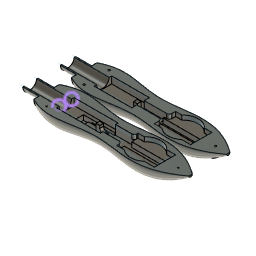
Fork V2 Fusion360 (Autodesk Fusion 360 design; units mm, degrees)
Autodesk Fusion 360 part; units mm, degrees
sketch "Sketch1" plane through (0, 0, 0) normal (0, 0, 1) x (1, 0, 0)
  line L0 (15.0107, 0) -> (130.0107, 0)
  line L1 (15.0107, 10.1439) -> (15.0107, 0)
  line L2 (130.0107, 1.3892) -> (130.0107, 0)
  spline S0 degree 5 poles (15.0107, 10.1439) (17.1655, 11.3215) (21.4632, 13.2587) (27.8735, 14.9106) (36.3471, 14.9335) (46.8266, 13.042) (57.2393, 11.1221) (67.6884, 10.6548) (78.3704, 11.8963) (89.578, 13.6649) (101.6455, 14.0909) (112.252, 11.6814) (120.8621, 7.5393) (126.9099, 3.6304) (130.0107, 1.3892) knots 0 0 0 0 0 0 0.1 0.2 0.3 0.4 0.5 0.6 0.7 0.8 0.9 1 1 1 1 1 1
  line L3 (5.0608, 4.7061) -> (24.9606, 15.5816)
  line L4 (117.8706, 10.1641) -> (142.1507, -7.3857)
  point P0 (63.5697, 11.0506)
  dimension "d2" = 115
  constraint horizontal L0
  constraint perpendicular L0 L1
  constraint perpendicular L0 L2
  constraint midpoint L1.start L3
  constraint midpoint L2.start L4
  measures "d2" distance of L0.start L0.end
revolve "Revolve1" add sketch "Sketch1" angle 360 about axis through (15.0107, 0, 0) along (1, 0, 0) makes body 1
sketch "Sketch2" plane through (0, 0, 0) normal (0, 0, 1) x (1, 0, 0)
sketch "Sketch3" plane through (15.0107, 0, 0) normal (-1, 0, 0) x (0, -1, 0)
  circle A0 centre (0, 0) radius 10.1439
  circle A1 centre (0, 0) radius 5
  circle A2 centre (0, 0) radius 6
  constraint coincident A0.centre A1.centre
extrude "Extrude1" add sketch "Sketch3" along normal blind 15 contours A2 bodies 1
extrude "Extrude2" cut 1 faces at (15.0107, 0.3379, -0.3642) along direction (1, 0, 0) blind 15 on bodies 1 bodies 1
split "Split1" by plane through (0, 0, 0) normal (0, 0, 1) bodies 1 makes body 2 at (53.0007, -11.0797, 4.6705)
move_body "Move1" bodies 2 to x (1, 0, 0) y (0, 1, 0) z (0, 0, 1) at (0, 0, 45)
sketch "Sketch4" plane through (0, 0, 0) normal (0, 0, 1) x (-1, 0, 0)
  line L0 (-15.0107, -6) -> (-0.0107, -6)
  line L1 (-0.0107, -6) -> (-0.0107, -5)
  line L2 (-0.0107, -5) -> (-30.0107, -5)
  line L3 (-30.0107, 5) -> (-0.0107, 5)
  line L4 (-0.0107, 5) -> (-0.0107, 6)
  line L5 (-0.0107, 6) -> (-15.0107, 6)
  line L6 (-15.0107, 6) -> (-15.0107, 10.1439)
  spline S0 degree 3 poles (-15.0107, 10.1439) (-17.2758, 11.3818) (-19.6235, 12.392) (-24.4058, 13.8233) (-26.7334, 14.2535) (-33.8193, 14.8563) (-38.417, 14.3623) (-51.6253, 12.321) (-59.2846, 10.4294) (-77.5088, 11.6941) (-83.806, 12.8904) (-95.9051, 13.7775) (-101.6068, 13.6874) (-114.9368, 10.4942) (-122.1312, 7.0845) (-130.0107, 1.3892) knots -19.403792 -19.403792 -19.403792 -19.403792 -17.868163 -17.868163 -16.437307 -16.437307 -13.646252 -13.646252 -8.493414 -8.493414 -5.456897 -5.456897 -2.916676 -2.916676 0 0 0 0
  line L7 (-130.0107, 1.3892) -> (-130.0107, -1.3892)
  spline S1 degree 5 poles (-15.0107, -10.1439) (-17.1655, -11.3215) (-21.4632, -13.2587) (-27.8735, -14.9106) (-36.3471, -14.9335) (-46.8266, -13.042) (-57.2393, -11.1221) (-67.6884, -10.6548) (-78.3704, -11.8963) (-89.578, -13.6649) (-101.6455, -14.0909) (-112.252, -11.6814) (-120.8621, -7.5393) (-126.9099, -3.6304) (-130.0107, -1.3892) knots 0 0 0 0 0 0 0.1 0.2 0.3 0.4 0.5 0.6 0.7 0.8 0.9 1 1 1 1 1 1
  line L8 (-15.0107, -10.1439) -> (-15.0107, -6)
move_body "Move2" bodies 2 to x (1, 0, 0) y (0, 1, 0) z (0, 0, 1) at (0, 65, 0)
sketch "Sketch5" plane through (0, 0, 0) normal (0, 0, 1) x (-1, 0, 0)
  line L0 (-30, -6) -> (-60, -6)
  line L1 (-60, -6) -> (-60, 6)
  line L2 (-60, 6) -> (-30, 6)
  line L3 (-30, 6) -> (-30, -6)
  constraint horizontal L0
  constraint vertical L1
  constraint horizontal L2
  constraint vertical L3
extrude "Extrude3" cut sketch "Sketch5" against normal blind 5.5 bodies 1
sketch "Sketch6" plane through (0, 0, 0) normal (0, 0, 1) x (1, 0, 0)
sketch "Sketch7" plane through (0, 0, -5.5) normal (0, 0, 1) x (-1, 0, 0)
  line L0 (-30, 6) -> (-60, 6)
  line L1 (-60, 6) -> (-60, -6)
  line L2 (-60, -6) -> (-30, -6)
  line L3 (-30, -6) -> (-30, 6)
  line L4 (-57, -1.5) -> (-59, -1.5)
  line L5 (-59, -1.5) -> (-59, 1.5)
  line L6 (-59, 1.5) -> (-57, 1.5)
  line L7 (-57, 1.5) -> (-57, -1.5)
  constraint horizontal L4
  constraint vertical L5
  constraint horizontal L6
  constraint vertical L7
extrude "Extrude4" add sketch "Sketch7" along normal blind 4 contours L4 L5 L6 L7 bodies 1
sketch "Sketch8" plane through (0, 0, 0) normal (0, 0, 1) x (-1, 0, 0)
  line L0 (-30, -5) -> (-30, -6)
  line L1 (-30, -6) -> (-60, -6)
  line L2 (-60, -6) -> (-60, 6)
  line L3 (-60, 6) -> (-30, 6)
  line L4 (-30, 6) -> (-30, 5)
  line L5 (-30, 5) -> (-0.0107, 5)
  line L6 (-0.0107, 5) -> (-0.0107, 6)
  line L7 (-0.0107, 6) -> (-15.0107, 6)
  line L8 (-15.0107, 6) -> (-15.0107, 10.1439)
  spline S0 degree 3 poles (-15.0107, 10.1439) (-17.2758, 11.3818) (-19.6235, 12.392) (-24.4058, 13.8233) (-26.7334, 14.2535) (-33.8193, 14.8563) (-38.417, 14.3623) (-51.6253, 12.321) (-59.2846, 10.4294) (-77.5088, 11.6941) (-83.806, 12.8904) (-95.9051, 13.7775) (-101.6068, 13.6874) (-114.9368, 10.4942) (-122.1312, 7.0845) (-130.0107, 1.3892) knots -19.403792 -19.403792 -19.403792 -19.403792 -17.868163 -17.868163 -16.437307 -16.437307 -13.646252 -13.646252 -8.493414 -8.493414 -5.456897 -5.456897 -2.916676 -2.916676 0 0 0 0
  line L9 (-130.0107, 1.3892) -> (-130.0107, -1.3892)
  spline S1 degree 5 poles (-15.0107, -10.1439) (-17.1655, -11.3215) (-21.4632, -13.2587) (-27.8735, -14.9106) (-36.3471, -14.9335) (-46.8266, -13.042) (-57.2393, -11.1221) (-67.6884, -10.6548) (-78.3704, -11.8963) (-89.578, -13.6649) (-101.6455, -14.0909) (-112.252, -11.6814) (-120.8621, -7.5393) (-126.9099, -3.6304) (-130.0107, -1.3892) knots 0 0 0 0 0 0 0.1 0.2 0.3 0.4 0.5 0.6 0.7 0.8 0.9 1 1 1 1 1 1
  line L10 (-15.0107, -10.1439) -> (-15.0107, -6)
  line L11 (-15.0107, -6) -> (-0.0107, -6)
  line L12 (-0.0107, -6) -> (-0.0107, -5)
  line L13 (-0.0107, -5) -> (-30, -5)
  line L14 (-60, -3) -> (-85, -3)
  line L15 (-85, -3) -> (-85, 3)
  line L16 (-85, 3) -> (-60, 3)
  line L17 (-60, 3) -> (-60, -3)
  constraint horizontal L14
  constraint vertical L15
  constraint horizontal L16
  constraint vertical L17
  constraint coincident L2 L14.start
extrude "Extrude5" cut sketch "Sketch8" against normal blind 2.5 contours L2 L14 L15 L16 L17 bodies 1
extrude "Extrude6" add 1 faces at (57.6667, 0.5, -1.5) along direction (0, 0, 1) blind 1 on bodies 1 bodies 1
sketch "Sketch9" plane through (0, 0, -5.5) normal (0, 0, 1) x (-1, 0, 0)
  line L0 (-57, 1.5) -> (-57, -1.5)
  line L1 (-57, -1.5) -> (-59, -1.5)
  line L2 (-59, -1.5) -> (-59, 1.5)
  line L3 (-59, 1.5) -> (-57, 1.5)
  line L4 (-30, 6) -> (-60, 6)
  line L5 (-60, 6) -> (-60, -6)
  line L6 (-60, -6) -> (-30, -6)
  line L7 (-30, -6) -> (-30, 6)
extrude "Extrude8" add 1 faces at (57, 0.5, -2.1667) along direction (-1, 0, 0) blind 2 on bodies 1 bodies 1
sketch "Sketch10" plane through (0, 0, 0) normal (0, 0, 1) x (-1, 0, 0)
  line L0 (-85, 3) -> (-60, 3)
  line L1 (-60, 3) -> (-60, 6)
  line L2 (-60, 6) -> (-30, 6)
  line L3 (-30, 6) -> (-30, 5)
  line L4 (-30, 5) -> (-0.0107, 5)
  line L5 (-0.0107, 5) -> (-0.0107, 6)
  line L6 (-0.0107, 6) -> (-15.0107, 6)
  line L7 (-15.0107, 6) -> (-15.0107, 10.1439)
  spline S0 degree 3 poles (-15.0107, 10.1439) (-17.2758, 11.3818) (-19.6235, 12.392) (-24.4058, 13.8233) (-26.7334, 14.2535) (-33.8193, 14.8563) (-38.417, 14.3623) (-51.6253, 12.321) (-59.2846, 10.4294) (-77.5088, 11.6941) (-83.806, 12.8904) (-95.9051, 13.7775) (-101.6068, 13.6874) (-114.9368, 10.4942) (-122.1312, 7.0845) (-130.0107, 1.3892) knots -19.403792 -19.403792 -19.403792 -19.403792 -17.868163 -17.868163 -16.437307 -16.437307 -13.646252 -13.646252 -8.493414 -8.493414 -5.456897 -5.456897 -2.916676 -2.916676 0 0 0 0
  line L8 (-130.0107, 1.3892) -> (-130.0107, -1.3892)
  spline S1 degree 5 poles (-15.0107, -10.1439) (-17.1655, -11.3215) (-21.4632, -13.2587) (-27.8735, -14.9106) (-36.3471, -14.9335) (-46.8266, -13.042) (-57.2393, -11.1221) (-67.6884, -10.6548) (-78.3704, -11.8963) (-89.578, -13.6649) (-101.6455, -14.0909) (-112.252, -11.6814) (-120.8621, -7.5393) (-126.9099, -3.6304) (-130.0107, -1.3892) knots 0 0 0 0 0 0 0.1 0.2 0.3 0.4 0.5 0.6 0.7 0.8 0.9 1 1 1 1 1 1
  line L9 (-15.0107, -10.1439) -> (-15.0107, -6)
  line L10 (-15.0107, -6) -> (-0.0107, -6)
  line L11 (-0.0107, -6) -> (-0.0107, -5)
  line L12 (-0.0107, -5) -> (-30, -5)
  line L13 (-30, -5) -> (-30, -6)
  line L14 (-30, -6) -> (-60, -6)
  line L15 (-60, -6) -> (-60, -3)
  line L16 (-60, -3) -> (-85, -3)
  line L17 (-85, -3) -> (-85, 3)
  line L18 (-80, -8) -> (-109, -8)
  line L19 (-109, -8) -> (-109, 9)
  line L20 (-109, 9) -> (-80, 9)
  line L21 (-80, 9) -> (-80, -8)
  dimension "d21" = 29
  dimension "d22" = 17
  constraint horizontal L18
  constraint vertical L19
  constraint horizontal L20
  constraint vertical L21
  measures "d21" distance of L18.start L18.end
  measures "d22" distance of L18.end L19.end
extrude "Extrude9" cut sketch "Sketch10" against normal blind 3.5 contours L0 L16 L17 L18 L19 L20 L21 bodies 1
extrude "Extrude10" cut 1 faces at (66.6667, 1, -2.5) along direction (0, 0, -1) blind 1 on bodies 1 bodies 1
sketch "Sketch11" plane through (0, 0, -3.5) normal (0, 0, 1) x (-1, 0, 0)
  line L0 (-80, -3) -> (-60, -3)
  line L1 (-60, -3) -> (-60, 3)
  line L2 (-60, 3) -> (-80, 3)
  line L3 (-80, 3) -> (-80, 9)
  line L4 (-80, 9) -> (-109, 9)
  line L5 (-109, 9) -> (-109, -8)
  line L6 (-109, -8) -> (-80, -8)
  line L7 (-80, -8) -> (-80, -3)
  line L8 (-76, -2) -> (-108, -2)
  line L9 (-108, -2) -> (-108, 2)
  line L10 (-108, 2) -> (-76, 2)
  line L11 (-76, 2) -> (-76, -2)
  constraint horizontal L8
  constraint vertical L9
  constraint horizontal L10
  constraint vertical L11
extrude "Extrude11" cut sketch "Sketch11" against normal blind 4 contours L8 L9 L10 L11 bodies 1
sketch "Sketch12" plane through (60, 0, 0) normal (-1, 0, 0) x (0, -1, 0)
  line L0 (-3, -3.5) -> (-3, 0)
  line L1 (-3, 0) -> (-6, 0)
  line L2 (-6, 0) -> (-6, -5.5)
  line L3 (-6, -5.5) -> (6, -5.5)
  line L4 (6, -5.5) -> (6, 0)
  line L5 (6, 0) -> (3, 0)
  line L6 (3, 0) -> (3, -3.5)
  line L7 (3, -3.5) -> (-3, -3.5)
  line L8 (-3, -3.5) -> (-3, -5.5)
  line L9 (3, -3.5) -> (3, -5.5)
  constraint coincident L0.start L7.end
  constraint coincident L3 L8.end
  constraint perpendicular L3 L8
  constraint coincident L6.end L7.start
  constraint coincident L3 L9.end
  constraint perpendicular L3 L9
extrude "Extrude12" cut sketch "Sketch12" against normal blind 16 contours L3 L7 L8 L9 bodies 1
copy_body "CopyPasteBodies1" bodies 1 makes body 3
move_body "Move3" bodies 3 to x (1, 0, 0) y (0, 1, 0) z (0, 0, 1) at (0, 40, 0)
sketch "Sketch13" plane through (0, 0, -5.5) normal (0, 0, 1) x (-1, 0, 0)
  line L0 (-40, -3.5) -> (-47, -3.5)
  line L1 (-47, -3.5) -> (-47, 3.5)
  line L2 (-47, 3.5) -> (-40, 3.5)
  line L3 (-40, 3.5) -> (-40, -3.5)
  dimension "d31" = 7
  dimension "d32" = 7
  constraint horizontal L0
  constraint vertical L1
  constraint horizontal L2
  constraint vertical L3
  measures "d31" distance of L0.start L0.end
  measures "d32" distance of L0.end L1.end
extrude "Extrude13" cut sketch "Sketch13" against normal blind 3 bodies 1
sketch "Sketch14" plane through (0, 0, -8.5) normal (0, 0, 1) x (-1, 0, 0)
  line L0 (-40, 3.5) -> (-47, 3.5)
  line L1 (-47, 3.5) -> (-47, -3.5)
  line L2 (-47, -3.5) -> (-40, -3.5)
  line L3 (-40, -3.5) -> (-40, 3.5)
  circle A0 centre (-43.5, 0) radius 2
  dimension "d35" = 4
  measures "d35" diameter of A0
extrude "Extrude14" cut sketch "Sketch14" against normal blind 6 contours A0 bodies 1
extrude "Extrude15" cut 1 faces at (43.5498, -2.9981, -8.5) along direction (0, 0, -1) blind 1 on bodies 1 bodies 1
extrude "Extrude16" cut 2 faces at (60, 4, -3.6667) (60, -4, -1.8333) along direction (1, 0, 0) blind 5 on bodies 1 bodies 1
sketch "Sketch15" plane through (0, 0, -5.5) normal (0, 0, 1) x (-1, 0, 0)
  line L0 (-47, -3.5) -> (-47, 3.5)
  line L1 (-47, 3.5) -> (-40, 3.5)
  line L2 (-40, 3.5) -> (-40, -3.5)
  line L3 (-40, -3.5) -> (-47, -3.5)
  line L4 (-30, 6) -> (-65, 6)
  line L5 (-65, 6) -> (-65, 3)
  line L6 (-65, 3) -> (-76, 3)
  line L7 (-76, 3) -> (-76, 2)
  line L8 (-76, 2) -> (-76, -2)
  line L9 (-76, -2) -> (-76, -3)
  line L10 (-76, -3) -> (-65, -3)
  line L11 (-65, -3) -> (-65, -6)
  line L12 (-65, -6) -> (-30, -6)
  line L13 (-30, -6) -> (-30, 6)
  line L14 (-59, 1.5) -> (-55, 1.5)
  line L15 (-55, 1.5) -> (-55, -1.5)
  line L16 (-55, -1.5) -> (-59, -1.5)
  line L17 (-59, -1.5) -> (-59, 1.5)
  line L18 (-47, 3.5) -> (-65.0368, 3.5)
  line L19 (-65.0368, 3.5) -> (-65.0368, 1.5)
  line L20 (-65.0368, 1.5) -> (-47, 1.5)
  line L21 (-47, 1.5) -> (-47, 3.5)
  line L22 (-47, -3.5) -> (-65.0096, -3.5)
  line L23 (-65.0096, -3.5) -> (-65.0096, -1.5274)
  line L24 (-65.0096, -1.5274) -> (-47, -1.5274)
  line L25 (-47, -1.5274) -> (-47, -3.5)
  constraint horizontal L18
  constraint vertical L19
  constraint horizontal L20
  constraint vertical L21
  constraint coincident L0.end L1.start
  constraint horizontal L22
  constraint vertical L23
  constraint horizontal L24
  constraint vertical L25
  constraint coincident L0.start L3.end
extrude "Extrude17" cut sketch "Sketch15" against normal blind 2 contours L0 L10 L11 L22 L23 L24 L25 | L0 L5 L6 L14 L18 L19 L20 L21 bodies 1
move_body "Move4" bodies 3 to x (1, 0, 0) y (0, 1, 0) z (0, 0, 1) at (0, -10, 0)
sketch "Sketch16" plane through (0, 0, 0) normal (0, 0, 1) x (-1, 0, 0)
  line L0 (-65, -6) -> (-65, -3)
  line L1 (-65, -3) -> (-80, -3)
  line L2 (-80, -3) -> (-80, -8)
  line L3 (-80, -8) -> (-109, -8)
  line L4 (-109, -8) -> (-109, 9)
  line L5 (-109, 9) -> (-80, 9)
  line L6 (-80, 9) -> (-80, 3)
  line L7 (-80, 3) -> (-65, 3)
  line L8 (-65, 3) -> (-65, 6)
  line L9 (-65, 6) -> (-30, 6)
  line L10 (-30, 6) -> (-30, 5)
  line L11 (-30, 5) -> (-0.0107, 5)
  line L12 (-0.0107, 5) -> (-0.0107, 6)
  line L13 (-0.0107, 6) -> (-15.0107, 6)
  line L14 (-15.0107, 6) -> (-15.0107, 10.1439)
  spline S0 degree 3 poles (-15.0107, 10.1439) (-17.2758, 11.3818) (-19.6235, 12.392) (-24.4058, 13.8233) (-26.7334, 14.2535) (-33.8193, 14.8563) (-38.417, 14.3623) (-51.6253, 12.321) (-59.2846, 10.4294) (-77.5088, 11.6941) (-83.806, 12.8904) (-95.9051, 13.7775) (-101.6068, 13.6874) (-114.9368, 10.4942) (-122.1312, 7.0845) (-130.0107, 1.3892) knots -19.403792 -19.403792 -19.403792 -19.403792 -17.868163 -17.868163 -16.437307 -16.437307 -13.646252 -13.646252 -8.493414 -8.493414 -5.456897 -5.456897 -2.916676 -2.916676 0 0 0 0
  line L15 (-130.0107, 1.3892) -> (-130.0107, -1.3892)
  spline S1 degree 5 poles (-15.0107, -10.1439) (-17.1655, -11.3215) (-21.4632, -13.2587) (-27.8735, -14.9106) (-36.3471, -14.9335) (-46.8266, -13.042) (-57.2393, -11.1221) (-67.6884, -10.6548) (-78.3704, -11.8963) (-89.578, -13.6649) (-101.6455, -14.0909) (-112.252, -11.6814) (-120.8621, -7.5393) (-126.9099, -3.6304) (-130.0107, -1.3892) knots 0 0 0 0 0 0 0.1 0.2 0.3 0.4 0.5 0.6 0.7 0.8 0.9 1 1 1 1 1 1
  line L16 (-15.0107, -10.1439) -> (-15.0107, -6)
  line L17 (-15.0107, -6) -> (-0.0107, -6)
  line L18 (-0.0107, -6) -> (-0.0107, -5)
  line L19 (-0.0107, -5) -> (-30, -5)
  line L20 (-30, -5) -> (-30, -6)
  line L21 (-30, -6) -> (-65, -6)
sketch "Sketch17" plane through (0, 0, 0) normal (0, 0, 1) x (-1, 0, 0)
  line L0 (-80, -21) -> (-80, -27)
  line L1 (-80, -27) -> (-60, -27)
  line L2 (-60, -27) -> (-60, -24)
  line L3 (-60, -24) -> (-30, -24)
  line L4 (-30, -24) -> (-30, -25)
  line L5 (-30, -25) -> (-0.0107, -25)
  line L6 (-0.0107, -25) -> (-0.0107, -24)
  line L7 (-0.0107, -24) -> (-15.0107, -24)
  line L8 (-15.0107, -24) -> (-15.0107, -19.8561)
  spline S0 degree 3 poles (-15.0107, -19.8561) (-17.2758, -18.6182) (-19.6235, -17.608) (-24.4058, -16.1767) (-26.7334, -15.7465) (-33.8193, -15.1437) (-38.417, -15.6377) (-51.6253, -17.679) (-59.2846, -19.5706) (-77.5088, -18.3059) (-83.806, -17.1096) (-95.9051, -16.2225) (-101.6068, -16.3126) (-114.9368, -19.5058) (-122.1312, -22.9155) (-130.0107, -28.6108) knots -19.403792 -19.403792 -19.403792 -19.403792 -17.868163 -17.868163 -16.437307 -16.437307 -13.646252 -13.646252 -8.493414 -8.493414 -5.456897 -5.456897 -2.916676 -2.916676 0 0 0 0
  line L9 (-130.0107, -28.6108) -> (-130.0107, -31.3892)
  spline S1 degree 5 poles (-15.0107, -40.1439) (-17.1655, -41.3215) (-21.4632, -43.2587) (-27.8735, -44.9106) (-36.3471, -44.9335) (-46.8266, -43.042) (-57.2393, -41.1221) (-67.6884, -40.6548) (-78.3704, -41.8963) (-89.578, -43.6649) (-101.6455, -44.0909) (-112.252, -41.6814) (-120.8621, -37.5393) (-126.9099, -33.6304) (-130.0107, -31.3892) knots 0 0 0 0 0 0 0.1 0.2 0.3 0.4 0.5 0.6 0.7 0.8 0.9 1 1 1 1 1 1
  line L10 (-15.0107, -40.1439) -> (-15.0107, -36)
  line L11 (-15.0107, -36) -> (-0.0107, -36)
  line L12 (-0.0107, -36) -> (-0.0107, -35)
  line L13 (-0.0107, -35) -> (-30, -35)
  line L14 (-30, -35) -> (-30, -36)
  line L15 (-30, -36) -> (-60, -36)
  line L16 (-60, -36) -> (-60, -33)
  line L17 (-60, -33) -> (-80, -33)
  line L18 (-80, -33) -> (-80, -38)
  line L19 (-80, -38) -> (-109, -38)
  line L20 (-109, -38) -> (-109, -21)
  line L21 (-109, -21) -> (-80, -21)
sketch "Sketch18" plane through (0, 0, 0) normal (0, 0, 1) x (-1, 0, 0)
  circle A0 centre (-120, 0) radius 0.5
  dimension "d44" = 1
  measures "d44" diameter of A0
extrude "Extrude18" cut sketch "Sketch18" against normal blind 5 bodies 1
sketch "Sketch19" plane through (0, 0, 0) normal (0, 0, 1) x (-1, 0, 0)
ref_plane "WorkPlane1" through (65.0107, 29.9083, -15) normal (0, 0, 1) x (-1, 0, 0)
sketch "Sketch20" plane through (0, 0, -15) normal (0, 0, 1) x (1, 0, 0)
  circle A0 centre (120, 30) radius 2.5
  dimension "d48" = 5
  measures "d48" diameter of A0
extrude "Extrude19" cut sketch "Sketch20" along normal blind 13 bodies 3
sketch "Sketch21" plane through (0, 0, -2) normal (0, 0, -1) x (1, 0, 0)
  circle A0 centre (120, -30) radius 2.5
  circle A1 centre (120, -30) radius 0.75
  dimension "d51" = 1.5
  constraint concentric A0 A1
  measures "d51" diameter of A1
extrude "Extrude20" cut sketch "Sketch21" against normal blind 10 contours A1 bodies 3
sketch "Sketch22" plane through (0, 0, 0) normal (0, 0, 1) x (-1, 0, 0)
  circle A0 centre (-25, 10) radius 0.5
  circle A1 centre (-25, -10) radius 0.5
  dimension "d54" = 1
  dimension "d55" = 1
  measures "d54" diameter of A0
  measures "d55" diameter of A1
extrude "Extrude21" cut sketch "Sketch22" against normal blind 5 contours A1 bodies 1
sketch "Sketch23" plane through (0, 0, 0) normal (0, 0, 1) x (-1, 0, 0)
  circle A0 centre (-25, 10) radius 0.5
  dimension "d58" = 1
  measures "d58" diameter of A0
extrude "Extrude22" cut sketch "Sketch23" against normal blind 5 bodies 1
sketch "Sketch24" plane through (0, 0, 0) normal (0, 0, 1) x (1, 0, 0)
ref_plane "WorkPlane2" through (65.0107, 29.9083, -15) normal (0, 0, 1) x (-1, 0, 0)
sketch "Sketch25" plane through (0, 0, -15) normal (0, 0, 1) x (1, 0, 0)
  circle A0 centre (25, 40) radius 2.25
  circle A1 centre (25, 20) radius 2.25
  dimension "d62" = 4.5
  dimension "d63" = 4.5
  measures "d62" diameter of A0
  measures "d63" diameter of A1
extrude "Extrude23" cut sketch "Sketch25" along normal blind 13 bodies 3
sketch "Sketch26" plane through (0, 0, -2) normal (0, 0, -1) x (1, 0, 0)
  circle A0 centre (25, -20) radius 2.25
  circle A1 centre (25, -20) radius 0.75
  dimension "d66" = 1.5
  constraint concentric A0 A1
  measures "d66" diameter of A1
extrude "Extrude24" cut sketch "Sketch26" against normal blind 10 contours A1 bodies 3
sketch "Sketch27" plane through (0, 0, -2) normal (0, 0, -1) x (1, 0, 0)
  circle A0 centre (25, -40) radius 2.25
  circle A1 centre (25, -40) radius 0.75
  dimension "d69" = 1.5
  constraint concentric A0 A1
  measures "d69" diameter of A1
extrude "Extrude25" cut sketch "Sketch27" against normal blind 10 contours A1 bodies 3
sketch "Sketch28" plane through (0, 0, 0) normal (0, 0, 1) x (-1, 0, 0)
ref_plane "WorkPlane3" through (92.5, -0.5, -3.5) normal (0, 0, 1) x (1, 0, 0)
sketch "Sketch29" plane through (0, 0, -3.5) normal (0, 0, 1) x (1, 0, 0)
ref_plane "WorkPlane4" through (92.5, -0.5, -3.5) normal (0, 0, 1) x (1, 0, 0)
sketch "Sketch30" plane through (0, 0, -3.5) normal (0, 0, 1) x (1, 0, 0)
  circle A0 centre (94, 0) radius 12
  dimension "d74" = 24
  measures "d74" diameter of A0
extrude "Extrude26" cut sketch "Sketch30" along normal blind 5 bodies 1
ref_plane "WorkPlane5" through (92.5, 29.5, -3.5) normal (0, 0, 1) x (1, 0, 0)
sketch "Sketch31" plane through (0, 0, -3.5) normal (0, 0, 1) x (1, 0, 0)
  circle A0 centre (94, 30) radius 12
  dimension "d78" = 24
  measures "d78" diameter of A0
extrude "Extrude27" cut sketch "Sketch31" along normal blind 10 bodies 3
extrude "Extrude28" cut 1 faces at (97.3333, 2, -5.5) along direction (0, 1, 0) blind 1 on bodies 1 bodies 1
extrude "Extrude29" cut 1 faces at (97.3333, -2, -5.5) along direction (0, -1, 0) blind 1 on bodies 1 bodies 1
extrude "Extrude30" cut 1 faces at (97.3333, 28, -5.5) along direction (0, -1, 0) blind 1 on bodies 3 bodies 3
extrude "Extrude31" cut 1 faces at (53.3333, -6, -1.8333) along direction (0, -1, 0) blind 1 on bodies 1 bodies 1
extrude "Extrude32" cut 1 faces at (41.6667, 6, -1.8333) along direction (0, 1, 0) blind 1 on bodies 1 bodies 1
extrude "Extrude33" cut 1 faces at (40, 36, -1.8333) along direction (0, 1, 0) blind 1 on bodies 3 bodies 3
extrude "Extrude34" cut 1 faces at (50, 24, -1.8333) along direction (0, -1, 0) blind 1 on bodies 3 bodies 3
extrude "Extrude35" cut 1 faces at (76, -1, -6.1667) along direction (-1, 0, 0) blind 13 on bodies 1 bodies 1
sketch "Sketch32" plane through (0, -3, 0) normal (0, 1, 0) x (-1, 0, 0)
  line L0 (-65, -7.5) -> (-65, 0)
  line L1 (-65, 0) -> (-80, 0)
  line L2 (-80, 0) -> (-80, -3.5)
  line L3 (-80, -3.5) -> (-108, -3.5)
  line L4 (-108, -3.5) -> (-108, -7.5)
  line L5 (-108, -7.5) -> (-65, -7.5)
  line L6 (-80, -3.5) -> (-80, -7.5)
  constraint coincident L2.end L3.start
  constraint coincident L5 L6.end
  constraint perpendicular L5 L6
extrude "Extrude36" cut sketch "Sketch32" against normal blind 2 contours L0 L1 L2 L5 L6 bodies 1
sketch "Sketch33" plane through (0, 3, 0) normal (0, -1, 0) x (1, 0, 0)
  line L0 (65, -7.5) -> (108, -7.5)
  line L1 (108, -7.5) -> (108, -3.5)
  line L2 (108, -3.5) -> (80, -3.5)
  line L3 (80, -3.5) -> (80, 0)
  line L4 (80, 0) -> (65, 0)
  line L5 (65, 0) -> (65, -7.5)
  line L6 (80, -3.5) -> (80, -7.5)
  constraint coincident L2.end L3.start
  constraint coincident L0 L6.end
  constraint perpendicular L0 L6
extrude "Extrude37" cut sketch "Sketch33" against normal blind 2 contours L0 L3 L4 L5 L6 bodies 1
extrude "Extrude38" cut 1 faces at (109, 2.3333, -1.1667) along direction (1, 0, 0) blind 1 on bodies 1 bodies 1
extrude "Extrude39" cut 1 faces at (108, 1, -6.1667) along direction (1, 0, 0) blind 2 on bodies 1 bodies 1
extrude "Extrude40" cut 1 faces at (55, 0.5, -2.1667) along direction (1, 0, 0) blind 1 on bodies 1 bodies 1
extrude "Extrude41" cut 1 faces at (55, 30.5, -2.1667) along direction (1, 0, 0) blind 1 on bodies 3 bodies 3
fillet "Fillet2" radius 3 1 edges at (59, 0, -5.5) on bodies 1
fillet "Fillet3" radius 2 2 edges at (80, 5, -1.75) (80, -5, -1.75) on bodies 1
fillet "Fillet4" radius 2 2 edges at (80, 33, -1.75) (80, 27, -1.75) on bodies 3
extrude "Extrude42" cut 1 faces at (42.3333, 3.5, -7.5) along direction (0, 1, 0) blind 1 on bodies 1 bodies 1
extrude "Extrude43" cut 1 faces at (42.3333, -3.5, -7.5) along direction (0, -1, 0) blind 1 on bodies 1 bodies 1
extrude "Extrude44" cut 1 faces at (0.0107, 24.3743, -0.5465) along direction (1, 0, 0) blind 2 on bodies 3 bodies 3
extrude "Extrude45" cut 1 faces at (0.0107, -5.6257, -0.5465) along direction (1, 0, 0) blind 2 on bodies 1 bodies 1
hidden bodies 2
